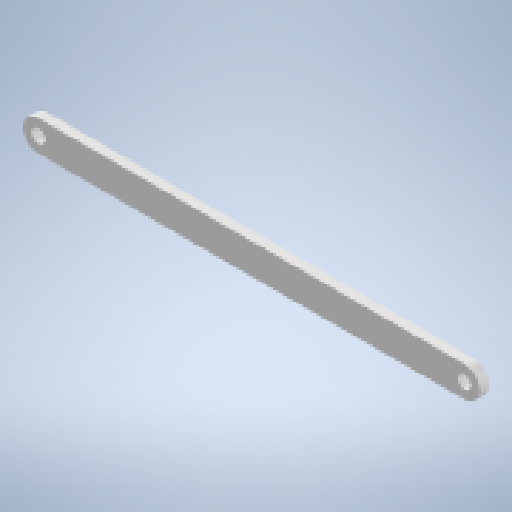
# Autodesk Inventor part: linkage
Saved by Autodesk Inventor 2024.1 (Build 281209000, 209)
## iProperties
Created: 2024-01-20
Part Number: linkage
Material: Generic
Document SubType Name: Modeling
Designer: luxsu
Density: 1 g/cm^3
Appearance: Default
Author: luxsu
Autodesk Inventor part; units mm, degrees
ref_plane "YZ Plane" through (0, 0, 0) normal (1, 0, 0) x (0, 1, 0)
ref_plane "XZ Plane" through (0, 0, 0) normal (0, 1, 0) x (-1, 0, 0)
ref_plane "XY Plane" through (0, 0, 0) normal (0, 0, 1) x (1, 0, 0)
sketch "Sketch1" plane through (0, 0, 0) normal (0, 0, 1) x (1, 0, 0)
  line L0 (0, 0) -> (135.404, 0) construction
  line L1 (0, -4.8511) -> (135.404, -4.8511)
  line L2 (135.404, 4.8511) -> (0, 4.8511)
  arc A0 (0, 4.8511) -> (0, -4.8511) centre (0, 0) ccw
  arc A1 (135.404, -4.8511) -> (135.404, 4.8511) centre (135.404, 0) ccw
  circle A2 centre (0, 0) radius 2.125
  circle A3 centre (135.404, 0) radius 2.125
  point P0 (67.702, 0)
  point P1 (0.702, -2.0057)
  point P2 (0.702, 2.0057)
  dimension "d0" = 135.404
  dimension "d1" = 4.25
  constraints: 8 end point, 4 centre point, 4 point on circle, 4 tangent, 2 coincident, 1 equal radius, 1 horizontal, 1 midpoint, 1 parallel
  measures "d0" distance of L0.end L0.start
  measures "d1" diameter of A2
extrude "Extrusion1" add sketch "Sketch1" along normal blind 3
body "Solid1"
